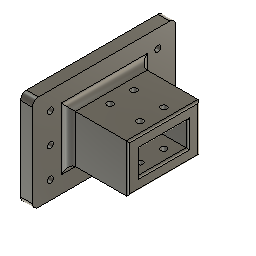
porta_etruso_20x40 v2 (Autodesk Fusion 360 design; units mm, degrees)
Autodesk Fusion 360 part; units mm, degrees
note: some values were not read from the file. Set by a fixed rule: which sketch regions a step uses.
sketch "Schizzo1" plane through (0, 0, 0) normal (1, 0, 0) x (0, 1, 0)
  line L0 (20.1, -10.1) -> (-20.1, -10.1)
  line L1 (-20.1, -10.1) -> (-20.1, 10.1)
  line L2 (-20.1, 10.1) -> (20.1, 10.1)
  line L3 (20.1, 10.1) -> (20.1, -10.1)
  line L4 (20.1, -10.1) -> (-20.1, 10.1) construction
  line L5 (-20.1, -10.1) -> (20.1, 10.1) construction
  line L6 (-60, -40) -> (60, -40)
  line L7 (60, -40) -> (60, 40)
  line L8 (60, 40) -> (-60, 40)
  line L9 (-60, 40) -> (-60, -40)
  line L10 (-60, -40) -> (60, 40) construction
  line L11 (60, -40) -> (-60, 40) construction
  dimension "d1" = 40.2
  dimension "d2" = 20.2
  dimension "d3" = 120
  dimension "d4" = 80
  constraint horizontal L0
  constraint perpendicular L0 L1
  constraint parallel L0 L2
  constraint parallel L1 L3
  constraint coincident L4 origin
  constraint coincident L5 origin
  constraint horizontal L6
  constraint perpendicular L6 L7
  constraint parallel L6 L8
  constraint parallel L7 L9
  constraint coincident L10 origin
  constraint coincident L11 origin
  measures "d1" distance of L1.end L2.end
  measures "d2" distance of L0.end L1.end
  measures "d3" distance of L7.end L8.end
  measures "d4" distance of L6.start L8.end
extrude "Estrusione1" add sketch "Schizzo1" along normal blind 10
sketch "Schizzo2" plane through (10, 0, 0) normal (1, 0, 0) x (0, 1, 0)
  line L0 (-20.1, 10.1) -> (20.1, 10.1)
  line L1 (20.1, 10.1) -> (20.1, -10.1)
  line L2 (20.1, -10.1) -> (-20.1, -10.1)
  line L3 (-20.1, -10.1) -> (-20.1, 10.1)
  line L4 (-60, 40) -> (-60, -40)
  line L5 (-60, -40) -> (60, -40)
  line L6 (60, -40) -> (60, 40)
  line L7 (60, 40) -> (-60, 40)
  line L8 (-20.1, -10.1) -> (20.1, -10.1)
  line L9 (20.1, -10.1) -> (20.1, 10.1)
  line L10 (20.1, 10.1) -> (-20.1, 10.1)
  line L11 (-20.1, 10.1) -> (-20.1, -10.1)
  line L12 (-20.1, -10.1) -> (20.1, 10.1) construction
  line L13 (20.1, -10.1) -> (-20.1, 10.1) construction
  line L14 (-30, -20) -> (30, -20)
  line L15 (30, -20) -> (30, 20)
  line L16 (30, 20) -> (-30, 20)
  line L17 (-30, 20) -> (-30, -20)
  line L18 (-30, -20) -> (30, 20) construction
  line L19 (30, -20) -> (-30, 20) construction
  dimension "d7" = 60
  dimension "d8" = 40
  constraint horizontal L8
  constraint perpendicular L8 L9
  constraint parallel L8 L10
  constraint parallel L9 L11
  constraint coincident L12 origin
  constraint coincident L13 origin
  constraint coincident L2.end L3.start
  constraint horizontal L14
  constraint perpendicular L14 L15
  constraint parallel L14 L16
  constraint parallel L15 L17
  constraint coincident L18 origin
  constraint coincident L19 origin
  measures "d7" distance of L15.end L16.end
  measures "d8" distance of L14.start L16.end
extrude "Estrusione2" add sketch "Schizzo2" along normal blind 50 contours L14 L15 L16 L17
sketch "Schizzo3" plane through (0, 0, -20) normal (0, 0, -1) x (1, 0, 0)
  line L0 (10, 30) -> (10, -30)
  line L1 (10, -30) -> (60, -30)
  line L2 (60, -30) -> (60, 30)
  line L3 (60, 30) -> (10, 30)
  line L4 (60, 0) -> (0, 0) construction
  line L5 (60, -10) -> (0, -10) construction
  circle A0 centre (50, -10) radius 2.5
  circle A1 centre (25, -10) radius 2.5
  circle A2 centre (50, 10) radius 2.5
  circle A3 centre (25, 10) radius 2.5
  point P0 (35, -10)
  dimension "d11" = 10
  dimension "d12" = 5
  dimension "d13" = 5
  dimension "d14" = 25
  dimension "d15" = 15
  dimension "d16" = 25
  constraint midpoint L2 L4.start
  constraint coincident L4.end origin
  constraint coincident L2 L5.start
  constraint perpendicular L0 L5
  constraint coincident L5 A0.centre
  constraint coincident L5 A1.centre
  constraint coincident L5 P0
  constraint symmetric L4 A0 A2
  constraint symmetric L4 A1 A3
  measures "d11" distance of L4 L5.start
  measures "d12" diameter of A0
  measures "d13" diameter of A1
  measures "d14" distance of A0.centre A1.centre
  measures "d15" distance of A0.centre P0
  measures "d16" distance of L2 P0
extrude "Estrusione3" cut sketch "Schizzo3" against normal blind 43 contours A0 | A1 | A2 | A3
sketch "Schizzo4" plane through (10, 0, 0) normal (1, 0, 0) x (0, 1, 0)
  line L0 (-30, 20) -> (30, 20)
  line L1 (30, 20) -> (30, -20)
  line L2 (30, -20) -> (-30, -20)
  line L3 (-30, -20) -> (-30, 20)
  line L4 (-60, 40) -> (-60, -40)
  line L5 (-60, -40) -> (60, -40)
  line L6 (60, -40) -> (60, 40)
  line L7 (60, 40) -> (-60, 40)
  line L8 (0, 40) -> (0, -40) construction
  line L9 (45, -40) -> (45, 40)
  circle A0 centre (45, 0) radius 2.5
  circle A1 centre (45, -25) radius 2.5
  circle A2 centre (45, 25) radius 2.5
  circle A3 centre (-45, -25) radius 2.5
  circle A4 centre (-45, 0) radius 2.5
  circle A5 centre (-45, 25) radius 2.5
  dimension "d19" = 5
  dimension "d20" = 5
  dimension "d21" = 5
  dimension "d22" = 25
  dimension "d23" = 25
  constraint midpoint L7 L8.start
  constraint midpoint L5 L8.end
  constraint coincident L5 L9.start
  constraint coincident L7 L9.end
  constraint perpendicular L7 L9
  constraint midpoint L9 A0.centre
  constraint coincident L9 A1.centre
  constraint coincident L9 A2.centre
  constraint symmetric L8 A0 A4
  constraint symmetric L8 A1 A3
  constraint symmetric L8 A2 A5
  measures "d19" diameter of A0
  measures "d20" diameter of A1
  measures "d21" diameter of A2
  measures "d22" distance of A0.centre A1.centre
  measures "d23" distance of A0.centre A2.centre
extrude "Estrusione4" cut sketch "Schizzo4" against normal blind 25 contours L9 A2 | L9 A2 | L9 A1 | L9 A1 | L9 A0 | L9 A0 | A3 | A4 | A5
fillet "Raccordo1" radius 5 4 edges at (5, 60, -40) (5, 60, 40) (5, -60, 40) (5, -60, -40)
fillet "Raccordo2" radius 6 4 edges at (10, 0, 20) (10, -30, 0) (10, 30, 0) (10, 0, -20)
fillet "Raccordo3" radius 1.5 8 edges at (60, 20.1, 0) (60, 0, -10.1) (60, 0, 10.1) (60, -20.1, 0) (60, -30, 0) (60, 0, 20) (60, 30, 0) (60, 0, -20)
